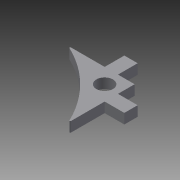
# Autodesk Inventor part: Gripper V 8.0 servo support bracket
Saved by Autodesk Inventor 2015 (Build 190159000, 159)
## iProperties
Created: 2015-06-24
Part Number: Gripper V 8.0 servo support bracket
Material: Generic
Document SubType Name: Modeling
Designer: Stackpole
Density: 1 g/cm^3
Appearance: Default
Author: Stackpole
Autodesk Inventor part; units mm, degrees
ref_plane "YZ Plane" through (0, 0, 0) normal (1, 0, 0) x (0, 1, 0)
ref_plane "XZ Plane" through (0, 0, 0) normal (0, 1, 0) x (-1, 0, 0)
ref_plane "XY Plane" through (0, 0, 0) normal (0, 0, 1) x (1, 0, 0)
sketch "Sketch1" plane through (0, 0, 0) normal (0, 0, 1) x (1, 0, 0)
  arc A0 (0, -20) -> (-20, 0) centre (-36.4575, -36.4575) ccw
  circle A1 centre (-4.5, -4.5) radius 2.5
  line L0 (-20, 0) -> (-9, 0)
  line L1 (-9, 0) -> (-9, 5.9)
  line L2 (-9, 5.9) -> (-5, 5.9)
  line L3 (-5, 5.9) -> (-5, 0)
  line L4 (-5, 0) -> (0, 0)
  line L5 (0, 0) -> (0, -5)
  line L6 (0, -5) -> (5.9, -5)
  line L7 (5.9, -5) -> (5.9, -9)
  line L8 (5.9, -9) -> (0, -9)
  line L9 (0, -9) -> (0, -20)
  dimension "d0" = 20
  dimension "d1" = 20
  dimension "d2" = 40
  dimension "d5" = 5
  dimension "d9" = 4
  dimension "d10" = 5.9
  dimension "d12" = 4.5
  dimension "d13" = 5.9
  dimension "d14" = 4
  dimension "d17" = 5
  dimension "d18" = 4.5
  dimension "d19" = 5
  constraints: 20 end point, 7 perpendicular, 2 centre point, 2 horizontal, 2 point on circle, 1 collinear, 1 point on line, 1 vertical
  measures "d0" distance of L4.end L9.end
  measures "d1" distance of L4.end L0.start
  measures "d2" radius of A0
  measures "d5" diameter of A1
  measures "d9" distance of L1.end L2.end
  measures "d10" distance of L0.end L1.end
  measures "d12" distance from line of L4 A1.centre
  measures "d13" distance of L5.end L6.end
  measures "d14" distance of L6.end L7.end
  measures "d17" distance between parallel lines of L6 L4
  measures "d18" distance from line of L5 A1.centre
  measures "d19" distance from line of L4.end L3
extrude "Extrusion1" add sketch "Sketch1" along normal blind 3
fillet "Fillet1" radius 0.2 2 edges at (0, -20, 1.5) (-20, 0, 1.5)
body "Solid1"
